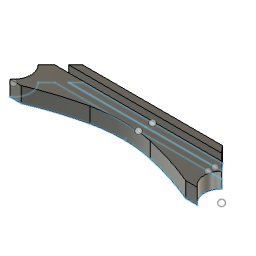
Finger1Section1P2V1 v2 (Autodesk Fusion 360 design; units mm, degrees)
Autodesk Fusion 360 part; units mm, degrees
sketch "Sketch1" plane through (0, 0, 0) normal (0, 0, 1) x (1, 0, 0)
  line L0 (4.507, 4) -> (5.507, 5)
  line L1 (2.3065, 1.7995) -> (3.507, 3)
  line L2 (2.071, -2) -> (3.6836, -2)
  arc A0 (2.071, -2) -> (2.3065, 1.7995) centre (0.571, 0) ccw
  line L3 (5.507, 5) -> (15.5594, 5)
  line L4 (25.5594, 5) -> (25.6118, 5)
  line L5 (4.507, 4) -> (15.5594, 4)
  line L6 (15.5594, 4) -> (4.507, 4)
  line L7 (27.507, 3) -> (25.5594, 3)
  line L8 (15.5594, 3) -> (3.507, 3)
  arc A1 (11.1884, 0.3961) -> (3.6836, -2) centre (20.507, -41.7412) ccw
  line L9 (28.7392, 1.7678) -> (27.507, 3)
  line L10 (25.5594, 4) -> (15.5594, 4)
  arc A2 (27.3304, -2) -> (19.8257, 0.3961) centre (10.507, -41.7412) ccw
  line L11 (27.507, 3) -> (15.5594, 3)
  line L12 (15.5594, 4) -> (26.507, 4)
  line L13 (25.6118, 5) -> (26.507, 4)
  line L14 (15.5594, 5) -> (25.6118, 5)
  line L15 (15.5594, 1.1297) -> (15.5594, 1.1174)
  line L16 (29.007, -2) -> (27.3304, -2)
  arc A3 (28.7392, 1.7678) -> (29.007, -2) centre (30.507, 0) ccw
  arc A4 (19.8257, 0.3961) -> (11.1884, 0.3961) centre (15.507, -19.1321) ccw
  dimension "d5" = 1
  dimension "d12" = 5
  dimension "d20" = 5
  dimension "d21" = 20
  constraint horizontal L5
  constraint horizontal L7
  constraint coincident L1.end L7
  constraint coincident L4.start L3
  constraint collinear L3 L4
  constraint collinear L7 L8
  constraint horizontal L10
  constraint horizontal L11
  constraint coincident L15.start A1
  constraint coincident L15.end A2
  constraint tangent A1 A4
  constraint tangent A2 A4
  measures "d5" distance of L5 L7
  measures "d12" diameter of A0
  measures "d20" diameter of A3
  measures "d21" radius of A4
extrude "Extrude3" add sketch "Sketch1" along normal blind 2.2 contours L1 L2 A0 L7 L8 A1 L9 A2 L11 L16 A3 A4 makes body 1
extrude "Extrude4" add sketch "Sketch1" along normal blind 2.2 separate body contours L0 L3 L4 L5 L6 L10 L12 L13 L14 makes body 2
